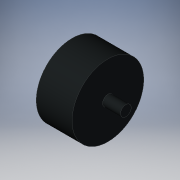
# Autodesk Inventor part: PRO10314 Rollenleiste Grundteil
Saved by Autodesk Inventor 2019 (Build 230136000, 136)
## iProperties
Created: 2023-08-22
Part Number: PRO10314 Rollenleiste Grundteil
Material: Generic
Catalog Web Link: www.cadenas.de
Description: PRO10314-Rollenleiste Grundteil
Vendor: ROBOTUNITS
Document SubType Name: Modeling
Designer: psAdmin
Manufacturer: ROBOTUNITS
Mass: 7.89914 g
Surface Area: 24.5987 cm^2
Volume: 7.89914 cm^3
Density: 1 g/cm^3
Appearance: PSOLRGB-127-135-137
Category: PARTsolutions
Company: ROBOTUNITS
Title: PRO10314 Rollenleiste Grundteil
Author: Cadenas PARTsolutions
Comments: Rollenleiste Grundteil
PSOL_IDENT_0: {$CADENAS_DATA/23d-libs/robotunits/mbs_pickstar/parts_materialbereitstellungssystem/pro_10314.prj},2
PSOL_IDENT_1: 04 {VTYP=3D},{NB=PRO10314 Rollenleiste Grundteil},{LINA=PRO10314 Rollenleiste Grundteil},{NN=PRO1031
PSOL_IDENT_2: 4},{DATE=25.04.2023 06:52:01},{GEOMDATE=14.02.2017 12:58:38},{VERSION=},{LINEID=10},{WBVAR=},{WBNUME
PSOL_IDENT_3: RIC=}  {NB=PRO10314 Rollenleiste Grundteil},{LINA=PRO10314 Rollenleiste Grundteil},{KT=DUMMY},{D=27.
PSOL_IDENT_4: 000}
NB: PRO10314 Rollenleiste Grundteil
NN: PRO10314
NT: Rollenleiste Grundteil
NBSYN: PRO10314 Rollenleiste Grundteil
LINA: PRO10314 Rollenleiste Grundteil
CATALOG: Robotunits
D: 27
SUPPLIER: ROBOTUNITS
ARTICLENO: PRO10314 Rollenleiste Grundteil
BOMINFO: PRO10314 Rollenleiste Grundteil
CREATOR: CADENAS GmbH
Autodesk Inventor part; units mm, degrees
ref_plane "YZ Plane" through (0, 0, 0) normal (1, 0, 0) x (0, 1, 0)
ref_plane "XZ Plane" through (0, 0, 0) normal (0, 1, 0) x (-1, 0, 0)
ref_plane "XY Plane" through (0, 0, 0) normal (0, 0, 1) x (1, 0, 0)
sketch "Sketch_1" plane through (0, 0, 0) normal (0, 0, 1) x (1, 0, 0)
  line L0 (50, 0) -> (-50, 0)
  line L1 (-13.5, 0) -> (-13.5, 2)
  line L2 (-13.5, 2) -> (-6.75, 2)
  line L3 (-6.75, 2) -> (-6.75, 13.5)
  line L4 (-6.75, 13.5) -> (6.75, 13.5)
  line L5 (6.75, 13.5) -> (6.75, 2)
  line L6 (6.75, 2) -> (13.5, 2)
  line L7 (13.5, 2) -> (13.5, 0)
  line L8 (13.5, 0) -> (-13.5, 0)
  constraints: 18 end point
revolve "Revolution1" add sketch "Sketch_1" angle 360 about axis through (50, 0, 0) along (1, 0, 0)
ref_plane "p1_XY" through (0, 0, 0) normal (1, 0, 0) x (0, 0, -1)
ref_plane "p1_YZ" through (0, 0, 0) normal (0, 0, -1) x (0, 1, 0)
ref_plane "p1_ZX" through (0, 0, 0) normal (0, 1, 0) x (1, 0, 0)
body "Solid1"
